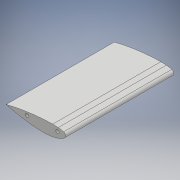
# Autodesk Inventor part: center flap
Saved by Autodesk Inventor 2018.3 (Build 223284000, 284)
## iProperties
Created: 2018-06-13
Part Number: center flap
Material: 一般
Document SubType Name: Modeling
Designer: ku_sk
Density: 1 g/cm^3
Appearance: 既定
Author: ku_sk
Autodesk Inventor part; units mm, degrees
ref_plane "YZ Plane" through (0, 0, 0) normal (1, 0, 0) x (0, 1, 0)
ref_plane "XZ Plane" through (0, 0, 0) normal (0, 1, 0) x (-1, 0, 0)
ref_plane "XY Plane" through (0, 0, 0) normal (0, 0, 1) x (1, 0, 0)
sketch "スケッチ1" plane through (0, 0, 0) normal (0, 1, 0) x (-1, 0, 0)
  arc A0 (101.6445, -27.9043) -> (207.0851, -9.0473) centre (48.6914, 572.4065) ccw projected
  arc A1 (76.001, -29.4031) -> (101.6445, -27.9043) centre (63.5114, 404.3974) ccw projected
  arc A2 (28.5134, -24.3454) -> (76.001, -29.4031) centre (70.891, 148.0818) ccw projected
  arc A3 (0.6182, -12.9849) -> (28.5134, -24.3454) centre (53.2617, 76.3513) ccw projected
  arc A4 (-7.3805, -6.2356) -> (0.6182, -12.9849) centre (16.4695, 13.9147) ccw projected
  arc A5 (-2.3661, 9.3678) -> (-7.3805, -6.2356) centre (0, 0) ccw projected
  arc A6 (17.4529, 12.5707) -> (-2.3661, 9.3678) centre (25.867, -102.4131) ccw projected
  arc A7 (37.3726, 13.7439) -> (17.4529, 12.5707) centre (68.6655, -687.2803) ccw projected
  arc A8 (207.0851, -9.0473) -> (37.3726, 13.7439) centre (17.751, -775.6364) ccw projected
  circle A9 centre (20.1088, -0.8575) radius 6 projected
  circle A10 centre (130.7072, -5.574) radius 6 projected
  point P0 (0, 0)
extrude "押し出し1" add sketch "スケッチ1" along normal mid plane 394
